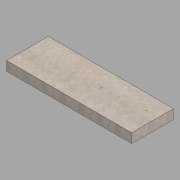
# Autodesk Inventor part: Bridge cap
Saved by Autodesk Inventor 2022 (Build 260153000, 153)
## iProperties
Created: 2021-10-21
Part Number: Bridge cap
Material: Limestone
Document SubType Name: Modeling
Designer: awelt
Density: 2.6 g/cm^3
Appearance: Kasota Gray
Mass: 118616 g
Surface Area: 12903.2 cm^2
Volume: 45621.6 cm^3
Author: awelt
Autodesk Inventor part; units mm, degrees
ref_plane "YZ Plane" through (0, 0, 0) normal (1, 0, 0) x (0, 1, 0)
ref_plane "XZ Plane" through (0, 0, 0) normal (0, 1, 0) x (-1, 0, 0)
ref_plane "XY Plane" through (0, 0, 0) normal (0, 0, 1) x (1, 0, 0)
sketch "Sketch1" plane through (0, 0, 0) normal (0, 1, 0) x (-1, 0, 0)
  line L0 (609.6, -203.2) -> (-609.6, -203.2)
  line L1 (-609.6, -203.2) -> (-609.6, 203.2)
  line L2 (-609.6, 203.2) -> (609.6, 203.2)
  line L3 (609.6, 203.2) -> (609.6, -203.2)
  line L4 (609.6, -203.2) -> (-609.6, 203.2) construction
  line L5 (-609.6, -203.2) -> (609.6, 203.2) construction
  point P0 (0, 0)
  dimension "d0" = 1219.2
  dimension "d1" = 406.4
  constraints: 12 end point, 2 midpoint, 2 parallel, 1 horizontal, 1 perpendicular
  measures "d0" distance of L1.end L2.end
  measures "d1" distance of L0.end L1.end
extrude "Extrusion1" add sketch "Sketch1" along normal blind 92.075
sketch "Sketch2" plane through (609.6, 0, 203.2) normal (1, 0, 0) x (0, 0, -1)
  line L0 (0, 0) -> (0, 92.075) projected
  line L1 (0, 87.3125) -> (6.35, 87.3125)
  line L2 (6.35, 87.3125) -> (6.35, 80.9625)
  line L3 (6.35, 80.9625) -> (0, 80.9625)
  line L4 (0, 80.9625) -> (0, 87.3125)
  line L5 (6.35, 68.2625) -> (0, 68.2625)
  line L6 (0, 68.2625) -> (0, 74.6125)
  line L7 (0, 74.6125) -> (6.35, 74.6125)
  line L8 (6.35, 74.6125) -> (6.35, 68.2625)
  line L9 (6.35, 55.5625) -> (0, 55.5625)
  line L10 (0, 55.5625) -> (0, 61.9125)
  line L11 (0, 61.9125) -> (6.35, 61.9125)
  line L12 (6.35, 61.9125) -> (6.35, 55.5625)
  line L13 (6.35, 42.8625) -> (0, 42.8625)
  line L14 (0, 42.8625) -> (0, 49.2125)
  line L15 (0, 49.2125) -> (6.35, 49.2125)
  line L16 (6.35, 49.2125) -> (6.35, 42.8625)
  line L17 (6.35, 30.1625) -> (0, 30.1625)
  line L18 (0, 30.1625) -> (0, 36.5125)
  line L19 (0, 36.5125) -> (6.35, 36.5125)
  line L20 (6.35, 36.5125) -> (6.35, 30.1625)
  line L21 (6.35, 17.4625) -> (0, 17.4625)
  line L22 (0, 17.4625) -> (0, 23.8125)
  line L23 (0, 23.8125) -> (6.35, 23.8125)
  line L24 (6.35, 23.8125) -> (6.35, 17.4625)
  line L25 (6.35, 4.7625) -> (0, 4.7625)
  line L26 (0, 4.7625) -> (0, 11.1125)
  line L27 (0, 11.1125) -> (6.35, 11.1125)
  line L28 (6.35, 11.1125) -> (6.35, 4.7625)
  point P0 (203.2, 0)
  point P1 (0, 4.7625)
  point P2 (0, 17.4625)
  point P3 (0, 30.1625)
  point P4 (0, 42.8625)
  point P5 (0, 55.5625)
  point P6 (0, 68.2625)
  point P7 (0, 80.9625)
  dimension "d4" = 6.35
  dimension "d5" = 6.35
  dimension "d6" = 4.7625
  dimension "d9" = 12.7
  dimension "d14" = 4.7625
  constraints: 56 end point, 2 parallel, 1 horizontal, 1 perpendicular, 1 point on line, 1 vertical, 48 other
  measures "d4" distance of L2.end L3.end
  measures "d5" distance of L1.end L2.end
  measures "d6" distance of L0.end L1.start
  measures "d9" distance of L2.end L5.start
  measures "d14" distance of L0.start L25.end
extrude "Extrusion2" [suppressed]
